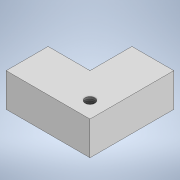
# Autodesk Inventor part: Footer
Saved by Autodesk Inventor 2022 (Build 260153000, 153)
## iProperties
Created: 2022-10-25
Part Number: Footer
Material: Ogólny
Document SubType Name: Modeling
Designer: kosak
Density: 1 g/cm^3
Appearance: Domyślna
Author: kosak
Autodesk Inventor part; units mm, degrees
ref_plane "YZ Plane" through (0, 0, 0) normal (1, 0, 0) x (0, 1, 0)
ref_plane "XZ Plane" through (0, 0, 0) normal (0, 1, 0) x (-1, 0, 0)
ref_plane "XY Plane" through (0, 0, 0) normal (0, 0, 1) x (1, 0, 0)
sketch "Szkic1" plane through (0, 0, 0) normal (0, 1, 0) x (-1, 0, 0)
  line L0 (0, 0) -> (30, 0)
  line L1 (30, 0) -> (30, 15)
  line L2 (30, 15) -> (0, 15)
  line L3 (0, 15) -> (0, 0)
  line L4 (0, 0) -> (15, 0)
  line L5 (15, 0) -> (15, -15)
  line L6 (15, -15) -> (0, -15)
  line L7 (0, -15) -> (0, 0)
  dimension "d0" = 30
  dimension "d1" = 15
  dimension "d2" = 15
  dimension "d3" = 15
  constraints: 16 end point, 4 parallel, 2 horizontal, 2 perpendicular
  measures "d0" distance of L2.end L1.end
  measures "d1" distance of L1.end L0.end
  measures "d2" distance of L5.end L6.end
  measures "d3" distance of L4.end L5.end
extrude "Wyciągnięcie proste1" add sketch "Szkic1" along normal blind 12
sketch "Szkic2" plane through (0, 0, 0) normal (0, -1, 0) x (1, 0, 0)
  line L0 (0, 9.242) -> (-5.758, 9.242)
  line L1 (-30, 15) -> (0, 15) projected
  line L2 (-5.758, 15) -> (-5.758, 9.242)
  circle A0 centre (-5.758, 9.242) radius 5
  point P0 (0, 0)
  dimension "d6" = 5.758
  dimension "d7" = 5.758
  dimension "d8" = 10
  constraints: 4 end point, 1 centre point, 1 coincident, 1 horizontal, 1 point on line, 1 vertical
  measures "d6" distance of L0.end L0.start
  measures "d7" distance of L2.start L0.end
  measures "d8" diameter of A0
extrude "Wyciągnięcie proste2" cut sketch "Szkic2" against normal blind 8
sketch "Szkic3" plane through (-5.758, 8, 9.242) normal (0, -1, 0) x (1, 0, 0)
  circle A0 centre (0, 0) radius 5 projected
  circle A1 centre (0, 0) radius 1.75
  point P0 (5.758, -9.242)
  dimension "d11" = 3.5
  constraints: 1 centre point, 1 coincident
  measures "d11" diameter of A1
extrude "Wyciągnięcie proste3" cut sketch "Szkic3" against normal blind 4 contours A1
thread "Gwint1" size "M3.5x0.6" class "6H" standard "ANSI Metric M Profile" full length
